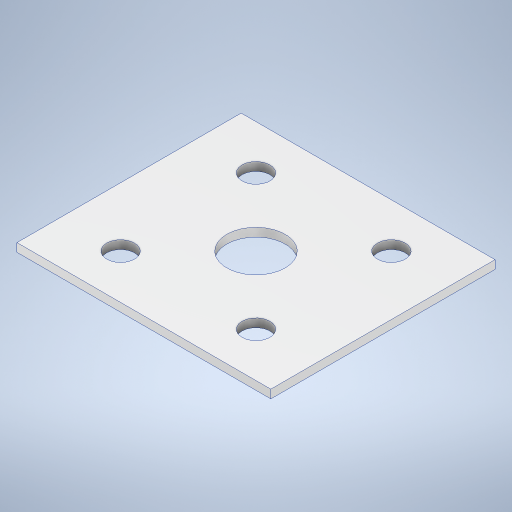
# Autodesk Inventor part: JGA25-370-bracket
Saved by Autodesk Inventor 2023 (Build 270158000, 158)
## iProperties
Created: 2022-05-10
Part Number: JGA25-370-bracket
Material: Aluminum 6061
Document SubType Name: Sheet Metal
Designer: Dan
Density: 2.7 g/cm^3
Sheet Metal Rule: Default_mm
Appearance: Aluminum - Flat
Author: Dan
Autodesk Inventor part; units mm, degrees
ref_plane "YZ Plane" through (0, 0, 0) normal (1, 0, 0) x (0, 1, 0)
ref_plane "XZ Plane" through (0, 0, 0) normal (0, 1, 0) x (-1, 0, 0)
ref_plane "XY Plane" through (0, 0, 0) normal (0, 0, 1) x (1, 0, 0)
sketch "Sketch14" plane through (0, 0, 0) normal (0, 1, 0) x (-1, 0, 0)
  line L0 (0, 0) -> (30, 0)
  line L1 (30, 0) -> (30, -26.5)
  line L2 (30, -26.5) -> (0, -26.5)
  line L3 (0, -26.5) -> (0, 0)
  circle A0 centre (15, -13.25) radius 3.45
  circle A1 centre (15, -13.25) radius 11.3137 construction
  circle A2 centre (23, -21.25) radius 1.65
  circle A3 centre (23, -5.25) radius 1.65
  circle A4 centre (7, -5.25) radius 1.65
  circle A5 centre (7, -21.25) radius 1.65
  line L4 (30, -13.25) -> (0, -13.25) construction
  dimension "d101" = 360
  dimension "d103" = 26.5
  dimension "d104" = 30
  dimension "d105" = 16
  dimension "d106" = 3.3
  dimension "d107" = 6.9
  measures "d103" distance of L0.end L1.end
  measures "d104" distance of L1.end L2.end
  measures "d105" distance of A3.centre A2.centre
  measures "d106" diameter of A2
  measures "d107" diameter of A0
extrude "Plate5" add sketch "Sketch14" along normal blind 1
equation "\"d108\" = Thickness"
equation "\"BendRadius\" = Thickness"
equation "\"BendReliefWidth\" = Thickness"
equation "\"BendReliefDepth\" = 0.5 * Thickness"
equation "\"CornerReliefSize\" = 4 * Thickness"
equation "\"MinimumRemnant\" = 2 * Thickness"
equation "\"TransitionRadius\" = BendRadius"
equation "\"JacobiRadiusSize\" = BendRadius"
equation "\"GapSize\" = Thickness"
equation "\"Thickness\" = 1"
body "Solid3"
